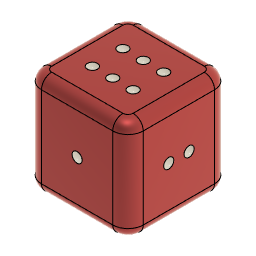
Basic Dice Cube v3 (Autodesk Fusion 360 design; units mm, degrees)
Autodesk Fusion 360 part; units mm, degrees
sketch "Sketch1" plane through (0, 0, 0) normal (0, 0, 1) x (1, 0, 0)
  line L0 (5, 5) -> (-5, 5)
  line L1 (-5, 5) -> (-5, -5)
  line L2 (-5, -5) -> (5, -5)
  line L3 (5, -5) -> (5, 5)
  line L4 (5, 5) -> (-5, -5) construction
  line L5 (-5, 5) -> (5, -5) construction
  dimension "d1" = 10
  dimension "d2" = 10
  constraint horizontal L0
  constraint perpendicular L0 L1
  constraint parallel L0 L2
  constraint parallel L1 L3
  constraint coincident L4 origin
  constraint coincident L5 origin
  measures "d1" distance of L1.end L2.end
  measures "d2" distance of L0.end L1.end
extrude "Extrude1" add sketch "Sketch1" along normal blind 10
sketch "Sketch2" plane through (0, -5, 0) normal (0, -1, 0) x (1, 0, 0)
  line L0 (-5, 0) -> (5, 0)
  line L1 (5, 0) -> (5, 10)
  line L2 (5, 10) -> (-5, 10)
  line L3 (-5, 10) -> (-5, 0)
  line L4 (-5, 5) -> (5, 5) construction
  circle A0 centre (0, 5) radius 0.5
  dimension "d5" = 1
  constraint midpoint L3 L4.start
  constraint midpoint L1 L4.end
  constraint midpoint L4 A0.centre
  measures "d5" diameter of A0
extrude "Extrude2" cut sketch "Sketch2" against normal blind 0.5 contours A0
sketch "Sketch3" plane through (5, 0, 0) normal (1, 0, 0) x (0, 1, 0)
  line L0 (-5, 0) -> (5, 0)
  line L1 (5, 0) -> (5, 10)
  line L2 (5, 10) -> (-5, 10)
  line L3 (-5, 10) -> (-5, 0)
  line L4 (-5, 5) -> (5, 5) construction
  line L5 (0, 5) -> (1, 5)
  line L6 (0, 5) -> (0, 3.5)
  circle A0 centre (1, 5) radius 0.5
  circle A1 centre (-1, 5) radius 0.5
  dimension "d8" = 1
  dimension "d9" = 1
  constraint midpoint L3 L4.start
  constraint midpoint L1 L4.end
  constraint midpoint L4 L5.start
  constraint parallel L4 L5
  constraint perpendicular L5 L6
  constraint coincident L5.end A0.centre
  constraint symmetric L6 A0 A1
  measures "d8" distance of L5.start L5.end
  measures "d9" diameter of A0
extrude "Extrude3" cut sketch "Sketch3" against normal blind 0.5 contours A0 | A1
sketch "Sketch4" plane through (0, 5, 0) normal (0, 1, 0) x (-1, 0, 0)
  line L0 (-5, 0) -> (5, 0)
  line L1 (5, 0) -> (5, 10)
  line L2 (5, 10) -> (-5, 10)
  line L3 (-5, 10) -> (-5, 0)
  line L4 (-5, 5) -> (5, 5) construction
  circle A0 centre (0, 5) radius 0.5
  line L5 (0, 5) -> (1.5, 5) construction
  circle A1 centre (1.5, 5) radius 0.5
  line L6 (0, 5) -> (0, 3) construction
  circle A2 centre (-1.5, 5) radius 0.5
  dimension "d12" = 1
  dimension "d13" = 1.5
  dimension "d14" = 1
  dimension "d15" = 2
  constraint midpoint L3 L4.start
  constraint midpoint L1 L4.end
  constraint midpoint L4 A0.centre
  constraint coincident A0.centre L5.start
  constraint parallel L4 L5
  constraint coincident L5.end A1.centre
  constraint perpendicular L4 L6
  constraint symmetric A1 L6 A2
  measures "d12" diameter of A0
  measures "d13" distance of A0.centre L5.end
  measures "d14" diameter of A1
  measures "d15" distance of A0.centre L6.end
extrude "Extrude4" cut sketch "Sketch4" against normal blind 0.5 contours A0 | A1 | A2
sketch "Sketch5" plane through (-5, 0, 0) normal (-1, 0, 0) x (0, -1, 0)
  line L0 (-5, 0) -> (5, 0)
  line L1 (5, 0) -> (5, 10)
  line L2 (5, 10) -> (-5, 10)
  line L3 (-5, 10) -> (-5, 0)
  line L4 (-5, 5) -> (5, 5) construction
  line L5 (1, 6) -> (-1, 6) construction
  line L6 (-1, 6) -> (-1, 4) construction
  line L7 (-1, 4) -> (1, 4) construction
  line L8 (1, 4) -> (1, 6) construction
  line L9 (1, 6) -> (-1, 4) construction
  line L10 (-1, 6) -> (1, 4) construction
  circle A0 centre (1, 6) radius 0.5
  circle A1 centre (-1, 6) radius 0.5
  circle A2 centre (1, 4) radius 0.5
  circle A3 centre (-1, 4) radius 0.5
  point P0 (0, 5)
  dimension "d18" = 2
  dimension "d19" = 2
  dimension "d20" = 1
  dimension "d21" = 1
  dimension "d22" = 1
  dimension "d23" = 1
  constraint midpoint L3 L4.start
  constraint midpoint L1 L4.end
  constraint horizontal L5
  constraint perpendicular L5 L6
  constraint parallel L5 L7
  constraint parallel L6 L8
  constraint coincident L9 P0
  constraint coincident L10 P0
  constraint midpoint L4 P0
  constraint coincident L5.start L8.end
  constraint coincident L5.end L6.start
  constraint coincident L7.end L8.start
  constraint coincident L6.end L7.start
  measures "d18" distance of L6.end L7.end
  measures "d19" distance of L5.end L6.end
  measures "d20" diameter of A0
  measures "d21" diameter of A1
  measures "d22" diameter of A2
  measures "d23" diameter of A3
extrude "Extrude5" cut sketch "Sketch5" against normal blind 0.5 contours A0 | A1 | A2 | A3
sketch "Sketch6" plane through (0, 0, 0) normal (0, 0, -1) x (1, 0, 0)
  line L0 (5, -5) -> (5, 5)
  line L1 (5, 5) -> (-5, 5)
  line L2 (-5, 5) -> (-5, -5)
  line L3 (-5, -5) -> (5, -5)
  line L4 (1.25, 1.25) -> (-1.25, 1.25) construction
  line L5 (-1.25, 1.25) -> (-1.25, -1.25) construction
  line L6 (-1.25, -1.25) -> (1.25, -1.25) construction
  line L7 (1.25, -1.25) -> (1.25, 1.25) construction
  line L8 (1.25, 1.25) -> (-1.25, -1.25) construction
  line L9 (-1.25, 1.25) -> (1.25, -1.25) construction
  circle A0 centre (0, 0) radius 0.5
  circle A1 centre (1.25, 1.25) radius 0.5
  circle A2 centre (-1.25, 1.25) radius 0.5
  circle A3 centre (1.25, -1.25) radius 0.5
  circle A4 centre (-1.25, -1.25) radius 0.5
  dimension "d26" = 2.5
  dimension "d27" = 2.5
  dimension "d28" = 1
  dimension "d29" = 1
  dimension "d30" = 1
  dimension "d31" = 1
  dimension "d32" = 1
  constraint horizontal L4
  constraint perpendicular L4 L5
  constraint parallel L4 L6
  constraint parallel L5 L7
  constraint coincident L8 A0.centre
  constraint coincident L9 A0.centre
  constraint coincident A0.centre origin
  constraint coincident L4.start L7.end
  constraint coincident L4.end L5.start
  constraint coincident L6.end L7.start
  constraint coincident L5.end L6.start
  measures "d26" distance of L5.end L6.end
  measures "d27" distance of L4.end L5.end
  measures "d28" diameter of A0
  measures "d29" diameter of A1
  measures "d30" diameter of A2
  measures "d31" diameter of A3
  measures "d32" diameter of A4
extrude "Extrude6" cut sketch "Sketch6" against normal blind 0.5 contours A0 | A1 | A2 | A3 | A4
sketch "Sketch7" plane through (0, 0, 10) normal (0, 0, 1) x (-1, 0, 0)
  line L0 (-5, 5) -> (-5, -5)
  line L1 (-5, -5) -> (5, -5)
  line L2 (5, -5) -> (5, 5)
  line L3 (5, 5) -> (-5, 5)
  line L4 (-2, -1.5) -> (2, -1.5) construction
  line L5 (2, -1.5) -> (2, 1.5) construction
  line L6 (2, 1.5) -> (-2, 1.5) construction
  line L7 (-2, 1.5) -> (-2, -1.5) construction
  line L8 (-2, -1.5) -> (2, 1.5) construction
  line L9 (2, -1.5) -> (-2, 1.5) construction
  circle A0 centre (2, -1.5) radius 0.5
  circle A1 centre (-2, -1.5) radius 0.5
  circle A2 centre (0, -1.5) radius 0.5
  line L10 (0, 0) -> (-1.2362, 0)
  circle A3 centre (2, 1.5) radius 0.5
  circle A4 centre (0, 1.5) radius 0.5
  circle A5 centre (-2, 1.5) radius 0.5
  dimension "d35" = 4
  dimension "d36" = 3
  dimension "d37" = 1
  dimension "d38" = 1
  dimension "d39" = 1
  constraint horizontal L4
  constraint perpendicular L4 L5
  constraint parallel L4 L6
  constraint parallel L5 L7
  constraint coincident L8 L10.start
  constraint coincident L9 L10.start
  constraint coincident L10.start origin
  constraint coincident L4.end L5.start
  constraint coincident L4.start L7.end
  constraint midpoint L4 A2.centre
  constraint horizontal L10
  constraint symmetric A0 L10 A3
  constraint symmetric A1 L10 A5
  constraint symmetric A2 L10 A4
  measures "d35" distance of L5.end L6.end
  measures "d36" distance of L4.end L5.end
  measures "d37" diameter of A0
  measures "d38" diameter of A1
  measures "d39" diameter of A2
extrude "Extrude7" cut sketch "Sketch7" against normal blind 0.5 contours A0 | A1 | A2 | A3 | A4 | A5
fillet "Fillet1" radius 1 8 edges at (5, 0, 10) (0, -5, 10) (-5, 0, 10) (0, 5, 10) (0, 5, 0) (5, 0, 0) (-5, 0, 0) (0, -5, 0)
fillet "Fillet1" radius 1.5 4 edges at (5, -5, 5) (5, 5, 5) (-5, 5, 5) (-5, -5, 5)
fillet "Fillet2" radius 0.5 21 edges at (4.5, -1.4662, 5.1808) (4.5, 0.5338, 5.1808) (-0.4662, -4.5, 5.1808) (-4.5, 1.4662, 6.1808) (-4.5, 1.4662, 4.1808) (-4.5, -0.5338, 6.1808) (-4.5, -0.5338, 4.1808) (0.4662, 4.5, 5.1808) (1.9662, 4.5, 5.1808) (-1.0338, 4.5, 5.1808) (-1.7162, 1.0692, 0.5) (-0.4662, -0.1808, 0.5) (-1.7162, -1.4308, 0.5) (0.7838, -1.4308, 0.5) (0.7838, 1.0692, 0.5) (2.4662, -1.6808, 9.5) (0.4662, -1.6808, 9.5) (-1.5338, -1.6808, 9.5) (0.4662, 1.3192, 9.5) (2.4662, 1.3192, 9.5) (-1.5338, 1.3192, 9.5)
